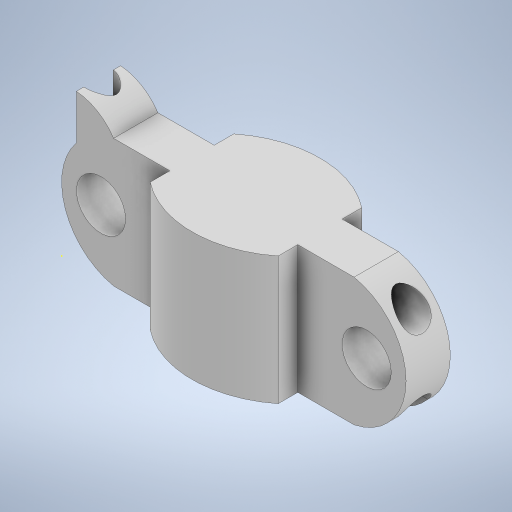
# Autodesk Inventor part: ProjEnAble_Finger_Philange
Saved by Autodesk Inventor 2023 (Build 270158000, 158)
## iProperties
Created: 2023-01-11
Part Number: ProjEnAble_Finger_Philange
Material: Generic
Document SubType Name: Modeling
Designer: jeron
Density: 1 g/cm^3
Appearance: Default
Author: jeron
Autodesk Inventor part; units mm, degrees
ref_plane "YZ Plane" through (0, 0, 0) normal (1, 0, 0) x (0, 1, 0)
ref_plane "XZ Plane" through (0, 0, 0) normal (0, 1, 0) x (-1, 0, 0)
sketch "Sketch1" plane through (0, 0, 0) normal (0, 0, 1) x (1, 0, 0)
  line L0 (0, 0) -> (35, 0)
  line L1 (35, 0) -> (35, 13)
  line L2 (35, 13) -> (0, 13)
  line L3 (0, 13) -> (0, 0)
  circle A0 centre (4, 6.5) radius 4
  circle A1 centre (4, 6.5) radius 2.5
  arc A2 (5.28125, 13) -> (5.28125, 0) centre (6.640625, 6.5) ccw
  line L4 (11, 13) -> (11, 0)
  circle A3 centre (31, 6.5) radius 4
  circle A4 centre (31, 6.5) radius 2.5
  arc A5 (29.71875, 0) -> (29.71875, 13) centre (28.359375, 6.5) ccw
  line L5 (24, 13) -> (24, 0)
  line L6 (9, 13) -> (11, 13)
  line L7 (26, 13) -> (24, 13)
  point P0 (0, 6.5)
  point P1 (29.71875, 13)
  point P2 (11, 0)
  point P3 (11, 13)
  dimension "d2" = 8
  dimension "d0" = 35
  dimension "d1" = 13
  dimension "d3" = 5
  dimension "d31" = 2
  dimension "d32" = 2
  constraints: 16 end point, 5 centre point, 5 point on circle, 4 point on line, 2 coincident, 2 parallel, 1 horizontal, 1 horizontal alignment, 1 midpoint, 1 perpendicular, 2 other
  measures "d0" distance of L2.end L1.end
  measures "d1" distance of L1.end L0.end
  measures "d3" diameter of A1
  measures "d31" distance of L6.start L6.end
  measures "d32" distance of L7.start L7.end
extrude "Extrusion1" add sketch "Sketch1" along normal mid plane 4.5 contours A0 | A2 L2 L4 L0 | A3 | L5 L2 A5 L0
extrude "Extrusion2" add sketch "Sketch1" along normal mid plane 13 contours L4 L2 L5 L0
sketch "Sketch2" plane through (29.71875, 13, 2.25) normal (0, 1, 0) x (1, 0, 0)
  line L0 (-18.71875, 0) -> (-24.4375, 0)
  line L1 (-18.71875, 0) -> (-18.71875, -2)
  line L2 (-24.4375, 4.5) -> (-18.71875, 4.5)
  line L3 (-18.71875, 4.5) -> (-18.71875, 6.5)
  line L4 (-18.71875, 8.75) -> (-18.71875, 4.5)
  line L5 (0, 4.5) -> (-5.71875, 4.5)
  line L6 (-5.71875, 4.5) -> (-5.71875, 6.5)
  line L7 (-5.71875, 0) -> (0, 0)
  line L8 (-5.71875, 0) -> (-5.71875, -2)
  line L9 (-5.71875, -4.25) -> (-5.71875, 0)
  line L10 (0, 0) -> (-5.71875, 0)
  line L11 (0, 0) -> (0, 4.5)
  line L12 (-5.71875, 4.5) -> (0, 4.5)
  line L13 (-5.71875, 4.5) -> (-5.71875, 8.75)
  line L14 (-18.71875, 8.75) -> (-5.71875, 8.75)
  line L15 (-18.71875, 8.75) -> (-18.71875, 4.5)
  line L16 (-24.4375, 4.5) -> (-18.71875, 4.5)
  line L17 (-24.4375, 4.5) -> (-24.4375, 0)
  line L18 (-18.71875, 0) -> (-24.4375, 0)
  line L19 (-18.71875, 0) -> (-18.71875, -4.25)
  line L20 (-5.71875, -4.25) -> (-18.71875, -4.25)
  line L21 (-5.71875, -4.25) -> (-5.71875, 0)
  arc A0 (-5.71875, 6.5) -> (-18.71875, 6.5) centre (-12.21875, -1.763889) ccw
  line L22 (-18.71875, 0) -> (-18.71875, -4.25)
  arc A1 (-18.71875, -2) -> (-5.71875, -2) centre (-12.21875, 6.263889) ccw
  point P0 (-29.71875, 2.25)
  point P1 (-12.21875, 8.75)
  point P2 (-12.21875, -4.25)
  point P3 (-18.71875, -2)
  dimension "d9" = 2
  dimension "d10" = 2
  dimension "d11" = 2
  dimension "d12" = 2
  constraints: 8 end point, 4 point on circle, 2 centre point, 2 point on line, 2 vertical, 1 tangent
  measures "d9" distance of L0.start L1.end
  measures "d10" distance of L2.end L3.end
  measures "d11" distance of L5.end L6.end
  measures "d12" distance of L7.start L8.end
ref_plane "Work Plane2" through (35, 6.5, -2.25) normal (1, 0, 0) x (0, 1, 0)
sketch "Sketch5" plane through (35, 6.5, -2.25) normal (1, 0, 0) x (0, 1, 0)
  line L0 (6.5, 1.5) -> (6.5, 3) projected
  circle A0 centre (4.25, 2.25) radius 1.5
  circle A1 centre (-4.25, 2.25) radius 1.5
  point P0 (-6.5, 2.25)
  dimension "d26" = 3
  constraints: 2 centre point
  measures "d26" diameter of A0
extrude "Extrusion7" cut sketch "Sketch5" against normal through all
sketch "Sketch6" plane through (5.28125, 0, -2.25) normal (0, -1, 0) x (1, 0, 0)
  spline S0 degree 5 poles (29.122577, 2.25) (29.122577, 2.418894) (29.111763, 2.588125) (29.090046, 2.75385) (29.056467, 2.912089) (28.971758, 3.174863) (28.925696, 3.283894) (28.870436, 3.382289) (28.805878, 3.467651) (28.670253, 3.598818) (28.601994, 3.648454) (28.52805, 3.686967) (28.449335, 3.714408) (28.273711, 3.751048) (28.175734, 3.757153) (28.074534, 3.751202) (27.971324, 3.734551) (27.652105, 3.654764) (27.432653, 3.560694) (27.217689, 3.436986) (27.008824, 3.286201) (26.75918, 3.039872) (26.697039, 2.971962) (26.638934, 2.899932) (26.586206, 2.823603) (26.489399, 2.653569) (26.446427, 2.557733) (26.415781, 2.457377) (26.400082, 2.354299) (26.400082, 2.09372) (26.435813, 1.937108) (26.504579, 1.794568) (26.589694, 1.66425) (26.789786, 1.420576) (26.906437, 1.307878) (27.030198, 1.207017) (27.157686, 1.117454) (27.402425, 0.970801) (27.518208, 0.911002) (27.635007, 0.860516) (27.751739, 0.820333) (27.971324, 0.765449) (28.074534, 0.748798) (28.175734, 0.742847) (28.273711, 0.748952) (28.450735, 0.785884) (28.530737, 0.813973) (28.605779, 0.853529) (28.674907, 0.904594) (28.783631, 1.011714) (28.826038, 1.062789) (28.86486, 1.119126) (28.900051, 1.180176) (29.012609, 1.413114) (29.068979, 1.606337) (29.104862, 1.816203) (29.122577, 2.033769) (29.122577, 2.25) knots 0 0 0 0 0 0 0.08399163 0.08399163 0.08399163 0.08399163 0.15051691 0.15051691 0.15051691 0.15051691 0.20678773 0.20678773 0.20678773 0.20678773 0.27091496 0.27091496 0.27091496 0.27091496 0.40360628 0.40360628 0.40360628 0.40360628 0.45015423 0.45015423 0.45015423 0.45015423 0.50155225 0.50155225 0.50155225 0.50155225 0.57856603 0.57856603 0.57856603 0.57856603 0.66015182 0.66015182 0.66015182 0.66015182 0.73091977 0.73091977 0.73091977 0.73091977 0.79460337 0.79460337 0.79460337 0.79460337 0.85143768 0.85143768 0.85143768 0.85143768 0.89302792 0.89302792 0.89302792 0.89302792 1 1 1 1 1 1
  spline S1 degree 5 poles (-1.962582, 2.25) (-1.962582, 2.354719) (-1.978408, 2.458196) (-2.009291, 2.55892) (-2.052576, 2.655082) (-2.149597, 2.824872) (-2.202108, 2.900742) (-2.259927, 2.972358) (-2.321733, 3.0399) (-2.571043, 3.285997) (-2.780002, 3.436882) (-2.994986, 3.560618) (-3.214535, 3.654747) (-3.533824, 3.734551) (-3.637034, 3.751202) (-3.738234, 3.757153) (-3.836211, 3.751048) (-4.013235, 3.714116) (-4.093237, 3.686027) (-4.168279, 3.646471) (-4.237407, 3.595406) (-4.463996, 3.372161) (-4.583598, 3.136777) (-4.65023, 2.851207) (-4.685077, 2.551066) (-4.685077, 1.946997) (-4.649777, 1.644964) (-4.582312, 1.357648) (-4.460904, 1.121833) (-4.232753, 0.901182) (-4.164494, 0.851546) (-4.09055, 0.813033) (-4.011835, 0.785592) (-3.836211, 0.748952) (-3.738234, 0.742847) (-3.637034, 0.748798) (-3.533824, 0.765449) (-3.214605, 0.845236) (-2.995153, 0.939306) (-2.780189, 1.063014) (-2.571324, 1.213799) (-2.32168, 1.460128) (-2.259539, 1.528038) (-2.201434, 1.600068) (-2.148706, 1.676397) (-2.051899, 1.846431) (-2.008927, 1.942267) (-1.978281, 2.042623) (-1.962582, 2.145701) (-1.962582, 2.25) knots 0 0 0 0 0 0 0.05146797 0.05146797 0.05146797 0.05146797 0.09764935 0.09764935 0.09764935 0.09764935 0.23003979 0.23003979 0.23003979 0.23003979 0.29400061 0.29400061 0.29400061 0.29400061 0.35108233 0.35108233 0.35108233 0.35108233 0.50001728 0.50001728 0.50001728 0.50001728 0.6499107 0.6499107 0.6499107 0.6499107 0.70602987 0.70602987 0.70602987 0.70602987 0.76998427 0.76998427 0.76998427 0.76998427 0.902318 0.902318 0.902318 0.902318 0.9487405 0.9487405 0.9487405 0.9487405 1 1 1 1 1 1
  line L0 (28.180615, 3.75) -> (-3.743115, 3.75)
  line L1 (28.180615, 0.75) -> (-3.743115, 0.75)
  line L2 (18.71875, 0) -> (18.71875, -4.25)
  line L3 (18.71875, 4.483177) -> (18.71875, 0)
  line L4 (5.71875, 4.5) -> (5.71875, 8.75)
  line L5 (5.71875, 4.5) -> (5.71875, 0)
  point P0 (-5.28125, 2.25)
  point P1 (20.71875, -2)
  point P2 (3.71875, 6.5)
  point P3 (5.71875, 0.75)
  point P4 (5.71875, 3.75)
  point P5 (18.71875, 3.75)
  point P6 (18.71875, 0.75)
  constraints: 4 end point, 1 perpendicular, 1 vertical, 4 other
sketch "Sketch6 outline for Extrusion8" plane through (5.28125, 0, -2.25) normal (0, -1, 0) x (1, 0, 0)
  line L0 (5.71875, 0.75) -> (5.71875, 3.75)
  line L1 (-3.743115, 0.75) -> (5.71875, 0.75)
  spline S0 degree 5 poles (-3.743115, 0.750005) (-3.682176, 0.750003) (-3.620097, 0.754459) (-3.557157, 0.763061) (-3.493637, 0.775494) (-3.214605, 0.845236) (-2.995153, 0.939306) (-2.780189, 1.063014) (-2.571324, 1.213799) (-2.32168, 1.460128) (-2.259539, 1.528038) (-2.201434, 1.600068) (-2.148706, 1.676397) (-2.051899, 1.846431) (-2.008927, 1.942267) (-1.978281, 2.042623) (-1.962582, 2.145701) (-1.962582, 2.25) knots 0 0 0 0 0 0 0.14574559 0.14574559 0.14574559 0.14574559 0.63721925 0.63721925 0.63721925 0.63721925 0.80962757 0.80962757 0.80962757 0.80962757 1 1 1 1 1 1
  spline S1 degree 5 poles (-1.962582, 2.25) (-1.962582, 2.354719) (-1.978408, 2.458196) (-2.009291, 2.55892) (-2.052576, 2.655082) (-2.149597, 2.824872) (-2.202108, 2.900742) (-2.259927, 2.972358) (-2.321733, 3.0399) (-2.571043, 3.285997) (-2.780002, 3.436882) (-2.994986, 3.560618) (-3.214535, 3.654747) (-3.493637, 3.724506) (-3.557157, 3.736939) (-3.620097, 3.745541) (-3.682176, 3.749997) (-3.743115, 3.749995) knots 0 0 0 0 0 0 0.19112679 0.19112679 0.19112679 0.19112679 0.36262179 0.36262179 0.36262179 0.36262179 0.85425494 0.85425494 0.85425494 0.85425494 1 1 1 1 1 1
  line L2 (5.71875, 3.75) -> (-3.743115, 3.75)
  line L3 (18.71875, 3.75) -> (18.71875, 0.75)
  line L4 (28.180615, 3.75) -> (18.71875, 3.75)
  spline S2 degree 5 poles (28.180615, 3.749995) (28.119676, 3.749997) (28.057597, 3.745541) (27.994657, 3.736939) (27.931137, 3.724506) (27.652105, 3.654764) (27.432653, 3.560694) (27.217689, 3.436986) (27.008824, 3.286201) (26.75918, 3.039872) (26.697039, 2.971962) (26.638934, 2.899932) (26.586206, 2.823603) (26.489399, 2.653569) (26.446427, 2.557733) (26.415781, 2.457377) (26.400082, 2.354299) (26.400082, 2.25) knots 0 0 0 0 0 0 0.14574559 0.14574559 0.14574559 0.14574559 0.63721924 0.63721924 0.63721924 0.63721924 0.80962756 0.80962756 0.80962756 0.80962756 1 1 1 1 1 1
  spline S3 degree 5 poles (26.400082, 2.25) (26.400082, 2.09372) (26.435813, 1.937108) (26.504579, 1.794568) (26.589694, 1.66425) (26.789786, 1.420576) (26.906437, 1.307878) (27.030198, 1.207017) (27.157686, 1.117454) (27.402425, 0.970801) (27.518208, 0.911002) (27.635007, 0.860516) (27.751739, 0.820333) (27.931137, 0.775494) (27.994657, 0.763061) (28.057597, 0.754459) (28.119676, 0.750003) (28.180615, 0.750005) knots 0 0 0 0 0 0 0.28688887 0.28688887 0.28688887 0.28688887 0.59080915 0.59080915 0.59080915 0.59080915 0.85443128 0.85443128 0.85443128 0.85443128 1 1 1 1 1 1
  line L5 (18.71875, 0.75) -> (28.180615, 0.75)
extrude "Extrusion8" cut sketch "Sketch6 outline for Extrusion8" against normal up to surface
extrude "Extrusion9" cut sketch "Sketch2" against normal through all contours A1 L20 L19 | A1 L9 L20 | L4 L14 A0 | L14 L13 A0
sketch "Sketch7" plane through (0, 0, 2.25) normal (0, 0, 1) x (1, 0, 0)
  point P0 (0, 0)
sketch "Sketch8" plane through (29.71875, 13, 2.25) normal (0, 1, 0) x (1, 0, 0)
  spline S0 degree 5 poles (-26.400082, 2.25) (-26.400082, 2.145281) (-26.415908, 2.041804) (-26.446791, 1.94108) (-26.490076, 1.844918) (-26.587097, 1.675128) (-26.639608, 1.599258) (-26.697427, 1.527642) (-26.759233, 1.4601) (-27.008543, 1.214003) (-27.217502, 1.063118) (-27.432486, 0.939382) (-27.652035, 0.845253) (-27.971324, 0.765449) (-28.074534, 0.748798) (-28.175734, 0.742847) (-28.273711, 0.748952) (-28.450735, 0.785884) (-28.530737, 0.813973) (-28.605779, 0.853529) (-28.674907, 0.904594) (-28.901496, 1.127839) (-29.021098, 1.363223) (-29.08773, 1.648793) (-29.122577, 1.948934) (-29.122577, 2.553003) (-29.087277, 2.855036) (-29.019812, 3.142352) (-28.898404, 3.378167) (-28.670253, 3.598818) (-28.601994, 3.648454) (-28.52805, 3.686967) (-28.449335, 3.714408) (-28.273711, 3.751048) (-28.175734, 3.757153) (-28.074534, 3.751202) (-27.971324, 3.734551) (-27.652105, 3.654764) (-27.432653, 3.560694) (-27.217689, 3.436986) (-27.008824, 3.286201) (-26.75918, 3.039872) (-26.697039, 2.971962) (-26.638934, 2.899932) (-26.586206, 2.823603) (-26.489399, 2.653569) (-26.446427, 2.557733) (-26.415781, 2.457377) (-26.400082, 2.354299) (-26.400082, 2.25) knots 0 0 0 0 0 0 0.05146797 0.05146797 0.05146797 0.05146797 0.09764935 0.09764935 0.09764935 0.09764935 0.23003979 0.23003979 0.23003979 0.23003979 0.29400061 0.29400061 0.29400061 0.29400061 0.35108233 0.35108233 0.35108233 0.35108233 0.50001728 0.50001728 0.50001728 0.50001728 0.6499107 0.6499107 0.6499107 0.6499107 0.70602987 0.70602987 0.70602987 0.70602987 0.76998427 0.76998427 0.76998427 0.76998427 0.902318 0.902318 0.902318 0.902318 0.9487405 0.9487405 0.9487405 0.9487405 1 1 1 1 1 1
  line L0 (-29.71875, 0) -> (-24.4375, 0)
  line L1 (-24.4375, 4.5) -> (-29.71875, 4.5)
  line L2 (-24.4375, 4.5) -> (-24.4375, 0)
  line L3 (-28.21875, 0.750712) -> (-28.21875, 0)
  line L4 (-28.21875, 4.5) -> (-23.21875, 4.5)
  line L5 (-28.21875, 3.749288) -> (-28.21875, 4.5)
  point P0 (-29.71875, 2.25)
  constraints: 4 end point, 1 perpendicular, 1 point on line, 1 vertical, 3 other
extrude "Extrusion10" add sketch "Sketch8" against normal up to surface contours S0 L5 L1 L2 L0 L3
extrude "Extrusion11" add sketch "Sketch8" along normal blind 2.25 contours S0 L5 L1 L2 L0 L3
sketch "Sketch9" plane through (0, 0, 2.25) normal (0, 0, 1) x (1, 0, 0)
  line L0 (5.28125, 0) -> (11, 0)
  line L1 (11, 0) -> (11, 13)
  line L2 (11, 13) -> (5.28125, 13)
  line L3 (5.28125, 13) -> (5.28125, 15.25)
  line L4 (1.5, 15.25) -> (5.28125, 15.25)
  line L5 (1.5, 10.703793) -> (1.5, 15.25)
  arc A0 (1.5, 10.703793) -> (5.28125, 0) centre (6.640625, 6.5) ccw
  circle A1 centre (4, 6.5) radius 2.5
  line L6 (5.28125, 13) -> (5.28125, 15.25)
  line L7 (5.28125, 13) -> (1.5, 13)
  arc A2 (5.28125, 13) -> (1.5, 15.25) centre (1.094634, 10.266459) ccw
  point P0 (0, 0)
  dimension "d39" = 5
  constraints: 2 end point, 2 point on circle, 1 centre point, 1 horizontal, 1 point on line
  measures "d39" radius of A2
extrude "Extrusion12" cut sketch "Sketch9" against normal through all contours A2 L4 L3
body "Solid1"
